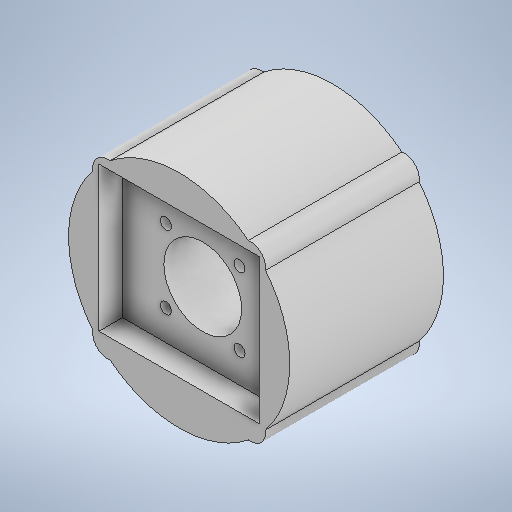
# Autodesk Inventor part: 2024_09_13_beam_combiner_blende_UHP_LED
Saved by Autodesk Inventor 2025.1 (Build 291241000, 241)
## iProperties
Created: 2023-11-21
Part Number: 2024_09_13_beam_combiner_blende_UHP_LED
Material: Generisch
Document SubType Name: Modeling
Designer: Daniel
Density: 1 g/cm^3
Appearance: Vorgabe
Author: Daniel
Autodesk Inventor part; units mm, degrees
ref_plane "YZ Plane" through (0, 0, 0) normal (1, 0, 0) x (0, 1, 0)
ref_plane "XZ Plane" through (0, 0, 0) normal (0, 1, 0) x (-1, 0, 0)
ref_plane "XY Plane" through (0, 0, 0) normal (0, 0, 1) x (1, 0, 0)
sketch "Sketch1" plane through (0, 0, 0) normal (0, 0, 1) x (1, 0, 0)
  circle A0 centre (0, 0) radius 11.25
  circle A1 centre (0, 0) radius 37.0304
  arc A2 (-32.7929, -17.201) -> (-31.2929, -19.799) centre (0, 0) ccw
  line L0 (-32.7929, -17.201) -> (-31.0547, -16.1974)
  line L1 (-32.7929, -17.201) -> (-31.0547, -16.1974)
  line L2 (-29.5547, -18.7955) -> (-31.2929, -19.799)
  line L3 (-31.2929, -19.799) -> (-29.5547, -18.7955)
  line L4 (-16.1974, -31.0547) -> (-17.201, -32.7929)
  line L5 (-17.201, -32.7929) -> (-16.1974, -31.0547)
  arc A3 (-19.799, -31.2929) -> (-17.201, -32.7929) centre (0, 0) ccw
  line L6 (-19.799, -31.2929) -> (-18.7955, -29.5547)
  line L7 (-19.799, -31.2929) -> (-18.7955, -29.5547)
  arc A4 (17.201, -32.7929) -> (19.799, -31.2929) centre (0, 0) ccw
  line L8 (17.201, -32.7929) -> (16.1974, -31.0547)
  line L9 (17.201, -32.7929) -> (16.1974, -31.0547)
  line L10 (18.7955, -29.5547) -> (19.799, -31.2929)
  line L11 (19.799, -31.2929) -> (18.7955, -29.5547)
  arc A5 (31.2929, -19.799) -> (32.7929, -17.201) centre (0, 0) ccw
  line L12 (31.2929, -19.799) -> (29.5547, -18.7955)
  line L13 (31.0547, -16.1974) -> (32.7929, -17.201)
  line L14 (32.7929, -17.201) -> (31.0547, -16.1974)
  line L15 (32.7929, 17.201) -> (31.0547, 16.1974)
  line L16 (32.7929, 17.201) -> (31.0547, 16.1974)
  arc A6 (32.7929, 17.201) -> (31.2929, 19.799) centre (0, 0) ccw
  line L17 (29.5547, 18.7955) -> (31.2929, 19.799)
  line L18 (31.2929, 19.799) -> (29.5547, 18.7955)
  line L19 (16.1974, 31.0547) -> (17.201, 32.7929)
  line L20 (17.201, 32.7929) -> (16.1974, 31.0547)
  line L21 (19.799, 31.2929) -> (18.7955, 29.5547)
  line L22 (19.799, 31.2929) -> (18.7955, 29.5547)
  line L23 (-17.201, 32.7929) -> (-16.1974, 31.0547)
  line L24 (-17.201, 32.7929) -> (-16.1974, 31.0547)
  line L25 (-18.7955, 29.5547) -> (-19.799, 31.2929)
  line L26 (-19.799, 31.2929) -> (-18.7955, 29.5547)
  arc A7 (-31.2929, 19.799) -> (-32.7929, 17.201) centre (0, 0) ccw
  line L27 (-31.2929, 19.799) -> (-29.5547, 18.7955)
  line L28 (-31.2929, 19.799) -> (-29.5547, 18.7955)
  line L29 (-31.0547, 16.1974) -> (-32.7929, 17.201)
  line L30 (-32.7929, 17.201) -> (-31.0547, 16.1974)
  arc A8 (-21.806, -27.4089) -> (-27.4089, -21.806) centre (-22.4506, -22.4506) ccw
  circle A9 centre (-31.75, 0) radius 5
  arc A10 (-3.9618, 34.8002) -> (-2.3096, 31.8679) centre (-22.4506, 22.4506) ccw
  circle A11 centre (-22.4506, 22.4506) radius 5
  circle A12 centre (22.4506, 22.4506) radius 5
  circle A13 centre (22.4506, 22.4506) radius 5
  arc A14 (-3.9618, -34.8002) -> (-1.7951, -38.6456) centre (22.4506, -22.4506) ccw
  circle A15 centre (22.4506, -22.4506) radius 5
  circle A16 centre (-22.4506, 22.4506) radius 4.75
  circle A17 centre (-22.4506, -22.4506) radius 4.75
  circle A18 centre (22.4506, -22.4506) radius 4.75
  circle A19 centre (22.4506, 22.4506) radius 4.75
  circle A20 centre (0, 0) radius 34.775
  circle A21 centre (0, 0) radius 36.75
  point P0 (0, 0)
  point P1 (0, 49.75)
  point P2 (27.1463, 21.7343)
  point P3 (21.7343, 27.1463)
  point P4 (-21.7343, 27.1463)
  point P5 (-27.1463, 21.7343)
  point P6 (-27.1463, -21.7343)
  point P7 (-21.7343, -27.1463)
  point P8 (21.7343, -27.1463)
  point P9 (27.1463, -21.7343)
  dimension "d6" = 70.05
  dimension "d8" = 74.0608
  dimension "d0" = 10
  dimension "d1" = 0.25
  dimension "d4" = 360
  dimension "d7" = 0.25
  dimension "d9" = 73.5
  constraints: 62 end point, 21 centre point, 18 point on circle, 15 collinear, 9 coincident, 8 other
  measures "d0" diameter of A11
  measures "d1" radial gap between concentric circles of A11 A16
  measures "d9" diameter of A21
extrude "Extrusion1" add sketch "Sketch1" along normal blind 48.3 contours A0 A10 | A9 A20 A11 A12 A15 A8 | A9 A20 A10 | A10 A20 A9 | A10 A0 | A20 A16 A11 | A8 A20 A17 | A20 A16 | A16 A20 | A20 A17 | A17 A20 | A15 A20 A18 | A20 A19 A12 | A20 A18 | A18 A20 | A20 A19 | A19 A20 picked at (-31.3962, -1.5997) picked at (-30.2693, 2.6951) picked at (-26.6756, 20.1619) picked at (20.1869, -26.6901) picked at (20.1869, 26.6901)
sketch "Skizze6" plane through (0, 0, 48.3) normal (0, 0, 1) x (1, 0, 0)
  circle A0 centre (0, 0) radius 12.225
  dimension "d33" = 24.45
  constraints: 1 centre point
  measures "d33" diameter of A0
extrude "Extrusion6" cut sketch "Skizze6" against normal through all
sketch "Skizze7" plane through (0, 0, 48.3) normal (0, 0, 1) x (1, 0, 0)
  line L0 (0, 0) -> (0, 1.75)
  line L1 (-25.23, 24.52) -> (25.23, 24.52)
  line L2 (25.23, 24.52) -> (25.23, -21.02)
  line L3 (25.23, -21.02) -> (-25.23, -21.02)
  line L4 (-25.23, -21.02) -> (-25.23, 24.52)
  line L5 (-25.23, 24.52) -> (25.23, -21.02) construction
  line L6 (25.23, 24.52) -> (-25.23, -21.02) construction
  dimension "d48" = 1.75
  dimension "d49" = 50.46
  dimension "d50" = 45.54
  constraints: 14 end point, 2 midpoint, 2 parallel, 1 horizontal, 1 perpendicular, 1 vertical
  measures "d48" distance of L0.start L0.end
  measures "d49" distance of L2.end L3.end
  measures "d50" distance of L1.end L2.end
extrude "Extrusion7" cut sketch "Skizze7" against normal blind 7.4
sketch "Skizze8" plane through (0, 0, 0) normal (0, 0, -1) x (-1, 0, 0)
  circle A0 centre (0, 0) radius 12.225 projected
  line L0 (-11.57, 11.47) -> (11.57, 11.47)
  line L1 (11.57, 11.57) -> (11.57, -11.57)
  line L2 (11.57, -11.57) -> (-11.57, -11.57)
  line L3 (-11.57, -11.57) -> (-11.57, 11.57)
  line L4 (-11.57, 11.57) -> (11.57, -11.57) construction
  line L5 (11.57, 11.57) -> (-11.57, -11.57) construction
  circle A1 centre (-11.57, 11.47) radius 1.75
  circle A2 centre (11.57, 11.47) radius 1.75
  circle A3 centre (11.57, -11.57) radius 1.75
  circle A4 centre (-11.57, -11.57) radius 1.75
  dimension "d40" = 23.14
  dimension "d41" = 23.14
  dimension "d42" = 3.5
  dimension "d43" = 3.5
  dimension "d44" = 3.5
  dimension "d45" = 3.5
  constraints: 12 end point, 5 coincident, 4 centre point, 2 midpoint, 2 parallel, 1 horizontal, 1 perpendicular
  measures "d40" distance of L1.end L2.end
  measures "d41" distance of L1.start L1.end
  measures "d42" diameter of A1
  measures "d43" diameter of A2
  measures "d44" diameter of A3
  measures "d45" diameter of A4
extrude "Extrusion8" cut sketch "Skizze8" against normal through all contours A2 L0 L1 | L1 L0 A2 | A3 L2 L1 | L1 L2 A3 | A1 L3 L0 | L0 L3 A1 | A4 L3 L2 | L2 L3 A4
sketch "Skizze9" plane through (0, 0, 0) normal (0, 0, -1) x (-1, 0, 0)
  circle A0 centre (-11.57, 11.47) radius 1.75 projected
  circle A1 centre (11.57, 11.47) radius 1.75 projected
  circle A2 centre (11.57, -11.57) radius 1.75 projected
  circle A3 centre (-11.57, -11.57) radius 1.75 projected
  circle A4 centre (-11.57, 11.47) radius 3.1
  circle A5 centre (11.57, 11.47) radius 3.1
  circle A6 centre (11.57, -11.57) radius 3.1
  circle A7 centre (-11.57, -11.57) radius 3.1
  point P0 (0, 0)
  dimension "d51" = 6.2
  dimension "d52" = 6.2
  dimension "d53" = 6.2
  dimension "d54" = 6.2
  constraints: 8 coincident, 4 centre point
  measures "d51" diameter of A4
  measures "d52" diameter of A5
  measures "d53" diameter of A6
  measures "d54" diameter of A7
extrude "Extrusion9" cut sketch "Skizze9" against normal blind 3.5 contours A0 | A1 | A2 | A3 | A4 | A5 | A6 | A7
body "Solid1"
